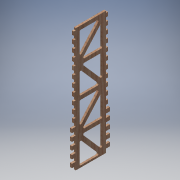
# Autodesk Inventor part: CrossBar4Alt
Saved by Autodesk Inventor 2019 (Build 230136000, 136)
## iProperties
Created: 2019-01-14
Part Number: CrossBar4Alt
Material: Wood (Birch)
Document SubType Name: Modeling
Designer: nxgam
Density: 0.55 g/cm^3
Appearance: Birch - Natural Polished
Author: nxgam
Autodesk Inventor part; units mm, degrees
ref_plane "YZ Plane" through (0, 0, 0) normal (1, 0, 0) x (0, 1, 0)
ref_plane "XZ Plane" through (0, 0, 0) normal (0, 1, 0) x (-1, 0, 0)
ref_plane "XY Plane" through (0, 0, 0) normal (0, 0, 1) x (1, 0, 0)
sketch "Sketch1" plane through (0, 0, 0) normal (1, 0, 0) x (0, 1, 0)
  line L0 (0, 0) -> (81.28, 0)
  line L1 (81.28, 0) -> (81.28, -91.44) construction
  line L2 (81.28, -91.44) -> (0, -91.44)
  line L3 (0, -91.44) -> (0, 0)
  line L4 (0, 0) -> (10.16, 0)
  line L5 (10.16, 0) -> (10.16, -5.08)
  line L6 (10.16, -5.08) -> (0, -5.08)
  line L7 (0, -5.08) -> (0, 0)
  line L8 (20.32, 0) -> (30.48, 0)
  line L9 (30.48, 0) -> (30.48, -5.08)
  line L10 (30.48, -5.08) -> (20.32, -5.08)
  line L11 (20.32, -5.08) -> (20.32, 0)
  line L12 (40.64, 0) -> (50.8, 0)
  line L13 (50.8, 0) -> (50.8, -5.08)
  line L14 (50.8, -5.08) -> (40.64, -5.08)
  line L15 (40.64, -5.08) -> (40.64, 0)
  line L16 (60.96, 0) -> (71.12, 0)
  line L17 (71.12, 0) -> (71.12, -5.08)
  line L18 (71.12, -5.08) -> (60.96, -5.08)
  line L19 (60.96, -5.08) -> (60.96, 0)
  line L20 (81.28, -45.72) -> (0, -45.72) construction
  line L21 (0, -91.44) -> (81.28, -91.44)
  line L22 (0, -91.44) -> (10.16, -91.44)
  line L23 (10.16, -91.44) -> (10.16, -86.36)
  line L24 (10.16, -86.36) -> (0, -86.36)
  line L25 (0, -86.36) -> (0, -91.44)
  line L26 (20.32, -91.44) -> (30.48, -91.44)
  line L27 (30.48, -91.44) -> (30.48, -86.36)
  line L28 (30.48, -86.36) -> (20.32, -86.36)
  line L29 (20.32, -86.36) -> (20.32, -91.44)
  line L30 (40.64, -91.44) -> (50.8, -91.44)
  line L31 (50.8, -91.44) -> (50.8, -86.36)
  line L32 (50.8, -86.36) -> (40.64, -86.36)
  line L33 (40.64, -86.36) -> (40.64, -91.44)
  line L34 (60.96, -91.44) -> (71.12, -91.44)
  line L35 (71.12, -91.44) -> (71.12, -86.36)
  line L36 (71.12, -86.36) -> (60.96, -86.36)
  line L37 (60.96, -86.36) -> (60.96, -91.44)
  line L38 (81.28, -86.36) -> (81.28, -91.44)
  line L39 (0, 0) -> (91.44, 0) construction
  line L40 (0, -91.44) -> (0, 0) construction
  line L41 (81.28, -10.16) -> (0, -10.16) construction
  line L42 (0, -10.16) -> (0, -81.28) construction
  line L43 (0, -81.28) -> (81.28, -81.28) construction
  line L44 (81.28, -81.28) -> (81.28, -10.16) construction
  line L45 (81.28, -10.16) -> (0, -81.28) construction
  line L46 (76.2, -28.3521) -> (76.2, -73.025)
  line L47 (73.025, -76.2) -> (21.9703, -76.2)
  line L48 (19.8795, -70.6356) -> (70.9342, -25.9627)
  arc A0 (76.2, -28.3521) -> (70.9342, -25.9627) centre (73.025, -28.3521) ccw
  arc A1 (73.025, -76.2) -> (76.2, -73.025) centre (73.025, -73.025) ccw
  arc A2 (19.8795, -70.6356) -> (21.9703, -76.2) centre (21.9703, -73.025) ccw
  line L49 (8.255, -15.24) -> (59.3097, -15.24)
  line L50 (61.4005, -20.8044) -> (10.3458, -65.4773)
  line L51 (5.08, -63.0879) -> (5.08, -18.415)
  arc A3 (61.4005, -20.8044) -> (59.3097, -15.24) centre (59.3097, -18.415) ccw
  arc A4 (5.08, -63.0879) -> (10.3458, -65.4773) centre (8.255, -63.0879) ccw
  arc A5 (8.255, -15.24) -> (5.08, -18.415) centre (8.255, -18.415) ccw
  line L52 (81.28, -45.72) -> (162.56, -45.72) construction
  line L53 (81.28, -10.16) -> (162.56, -10.16) construction
  line L54 (162.56, -81.28) -> (81.28, -81.28) construction
  line L55 (81.28, -10.16) -> (162.56, -81.28) construction
  line L56 (86.36, -28.3521) -> (86.36, -73.025)
  line L57 (89.535, -76.2) -> (140.5897, -76.2)
  line L58 (142.6805, -70.6356) -> (91.6258, -25.9627)
  arc A6 (91.6258, -25.9627) -> (86.36, -28.3521) centre (89.535, -28.3521) ccw
  arc A7 (86.36, -73.025) -> (89.535, -76.2) centre (89.535, -73.025) ccw
  arc A8 (140.5897, -76.2) -> (142.6805, -70.6356) centre (140.5897, -73.025) ccw
  line L59 (154.305, -15.24) -> (103.2503, -15.24)
  line L60 (101.1595, -20.8044) -> (152.2142, -65.4773)
  line L61 (157.48, -63.0879) -> (157.48, -18.415)
  arc A9 (103.2503, -15.24) -> (101.1595, -20.8044) centre (103.2503, -18.415) ccw
  arc A10 (152.2142, -65.4773) -> (157.48, -63.0879) centre (154.305, -63.0879) ccw
  arc A11 (157.48, -18.415) -> (154.305, -15.24) centre (154.305, -18.415) ccw
  line L62 (132.08, -86.36) -> (121.92, -86.36)
  line L63 (101.6, -86.36) -> (101.6, -91.44)
  line L64 (101.6, -91.44) -> (111.76, -91.44)
  line L65 (111.76, -91.44) -> (111.76, -86.36)
  line L66 (111.76, -86.36) -> (101.6, -86.36)
  line L67 (91.44, -86.36) -> (81.28, -86.36)
  line L68 (91.44, -91.44) -> (91.44, -86.36)
  line L69 (81.28, -91.44) -> (91.44, -91.44)
  line L70 (81.28, -91.44) -> (162.56, -91.44)
  line L71 (162.56, -91.44) -> (81.28, -91.44)
  line L72 (81.28, -81.28) -> (162.56, -81.28) construction
  line L73 (81.28, -10.16) -> (81.28, -81.28) construction
  line L74 (162.56, 0) -> (162.56, -91.44)
  line L75 (81.28, -91.44) -> (81.28, 0) construction
  line L76 (81.28, -91.44) -> (81.28, 0) construction
  line L77 (81.28, 0) -> (162.56, 0)
  line L78 (81.28, 0) -> (91.44, 0)
  line L79 (91.44, 0) -> (91.44, -5.08)
  line L80 (81.28, -5.08) -> (81.28, 0)
  line L81 (91.44, -5.08) -> (81.28, -5.08)
  line L82 (111.76, -5.08) -> (101.6, -5.08)
  line L83 (101.6, 0) -> (111.76, 0)
  line L84 (101.6, -5.08) -> (101.6, 0)
  line L85 (111.76, 0) -> (111.76, -5.08)
  line L86 (132.08, -5.08) -> (121.92, -5.08)
  line L87 (132.08, 0) -> (132.08, -5.08)
  line L88 (121.92, -5.08) -> (121.92, 0)
  line L89 (121.92, 0) -> (132.08, 0)
  line L90 (142.24, -5.08) -> (142.24, 0)
  line L91 (152.4, -5.08) -> (142.24, -5.08)
  line L92 (142.24, 0) -> (152.4, 0)
  line L93 (152.4, 0) -> (152.4, -5.08)
  line L94 (81.28, -86.36) -> (81.28, -91.44)
  line L95 (152.4, -86.36) -> (142.24, -86.36)
  line L96 (142.24, -91.44) -> (152.4, -91.44)
  line L97 (162.56, -86.36) -> (162.56, -91.44)
  line L98 (132.08, -91.44) -> (132.08, -86.36)
  line L99 (81.28, 0) -> (172.72, 0) construction
  line L100 (152.4, -91.44) -> (152.4, -86.36)
  line L101 (121.92, -86.36) -> (121.92, -91.44)
  line L102 (142.24, -86.36) -> (142.24, -91.44)
  line L103 (162.56, -81.28) -> (162.56, -10.16) construction
  line L104 (121.92, -91.44) -> (132.08, -91.44)
  line L105 (162.56, -10.16) -> (81.28, -10.16) construction
  line L106 (243.84, -81.28) -> (162.56, -81.28) construction
  line L107 (162.56, -45.72) -> (243.84, -45.72) construction
  line L108 (162.56, -10.16) -> (243.84, -81.28) construction
  line L109 (162.56, -10.16) -> (243.84, -10.16) construction
  line L110 (162.56, 0) -> (0, 0)
  line L111 (0, 0) -> (0, -91.44)
  line L112 (0, -91.44) -> (162.56, -91.44)
  line L113 (162.56, -91.44) -> (162.56, 0)
  line L114 (162.56, -91.44) -> (162.56, 0)
  line L115 (203.2, -86.36) -> (203.2, -91.44)
  line L116 (243.84, -45.72) -> (162.56, -45.72) construction
  line L117 (162.56, -81.28) -> (243.84, -81.28) construction
  line L118 (243.84, -10.16) -> (162.56, -81.28) construction
  line L119 (243.84, -10.16) -> (162.56, -10.16) construction
  line L120 (162.56, 0) -> (243.84, 0)
  line L121 (243.84, -91.44) -> (243.84, 0) construction
  line L122 (243.84, 0) -> (243.84, -91.44) construction
  line L123 (243.84, -91.44) -> (243.84, 0) construction
  line L124 (243.84, -91.44) -> (162.56, -91.44)
  line L125 (162.56, -91.44) -> (243.84, -91.44)
  line L126 (162.56, 0) -> (254, 0) construction
  line L127 (325.12, 0) -> (162.56, 0)
  line L128 (162.56, -91.44) -> (325.12, -91.44)
  line L129 (233.68, -91.44) -> (233.68, -86.36)
  line L130 (235.585, -76.2) -> (184.5303, -76.2)
  line L131 (223.52, -86.36) -> (223.52, -91.44)
  line L132 (243.84, -81.28) -> (243.84, -10.16) construction
  line L133 (193.04, 0) -> (193.04, -5.08)
  line L134 (193.04, -91.44) -> (193.04, -86.36)
  line L135 (193.04, -5.08) -> (182.88, -5.08)
  line L136 (193.04, -86.36) -> (182.88, -86.36)
  line L137 (182.88, -86.36) -> (182.88, -91.44)
  line L138 (172.72, 0) -> (172.72, -5.08)
  line L139 (162.56, -91.44) -> (162.56, 0) construction
  line L140 (162.56, 0) -> (172.72, 0)
  line L141 (162.56, -5.08) -> (162.56, 0)
  line L142 (162.56, -86.36) -> (162.56, -91.44)
  line L143 (172.72, -86.36) -> (162.56, -86.36)
  line L144 (172.72, -5.08) -> (162.56, -5.08)
  line L145 (162.56, -10.16) -> (162.56, -81.28) construction
  line L146 (223.52, -5.08) -> (223.52, 0)
  line L147 (233.68, -5.08) -> (223.52, -5.08)
  line L148 (223.52, 0) -> (233.68, 0)
  line L149 (233.68, 0) -> (233.68, -5.08)
  arc A12 (238.76, -28.3521) -> (233.4942, -25.9627) centre (235.585, -28.3521) ccw
  line L150 (182.88, -5.08) -> (182.88, 0)
  line L151 (254, -86.36) -> (243.84, -86.36)
  line L152 (264.16, -86.36) -> (264.16, -91.44)
  line L153 (264.16, -91.44) -> (274.32, -91.44)
  line L154 (294.64, -86.36) -> (284.48, -86.36)
  line L155 (316.865, -15.24) -> (265.8103, -15.24)
  line L156 (274.32, -86.36) -> (264.16, -86.36)
  line L157 (274.32, -91.44) -> (274.32, -86.36)
  line L158 (305.2405, -70.6356) -> (254.1858, -25.9627)
  arc A13 (248.92, -73.025) -> (252.095, -76.2) centre (252.095, -73.025) ccw
  line L159 (243.84, -10.16) -> (243.84, -81.28) construction
  arc A14 (265.8103, -15.24) -> (263.7195, -20.8044) centre (265.8103, -18.415) ccw
  line L160 (274.32, -5.08) -> (264.16, -5.08)
  line L161 (274.32, 0) -> (274.32, -5.08)
  line L162 (252.095, -76.2) -> (303.1497, -76.2)
  line L163 (263.7195, -20.8044) -> (314.7742, -65.4773)
  line L164 (325.12, -81.28) -> (243.84, -81.28) construction
  line L165 (243.84, -81.28) -> (325.12, -81.28) construction
  line L166 (243.84, -10.16) -> (325.12, -81.28) construction
  line L167 (243.84, -45.72) -> (325.12, -45.72) construction
  line L168 (243.84, -10.16) -> (325.12, -10.16) construction
  line L169 (325.12, -10.16) -> (243.84, -10.16) construction
  line L170 (243.84, 0) -> (325.12, 0)
  line L171 (243.84, 0) -> (335.28, 0) construction
  line L172 (320.04, -63.0879) -> (320.04, -18.415)
  line L173 (325.12, -91.44) -> (325.12, 0)
  line L174 (325.12, 0) -> (325.12, -91.44)
  arc A15 (314.7742, -65.4773) -> (320.04, -63.0879) centre (316.865, -63.0879) ccw
  line L175 (325.12, -91.44) -> (243.84, -91.44)
  line L176 (243.84, -91.44) -> (325.12, -91.44)
  line L177 (284.48, -86.36) -> (284.48, -91.44)
  line L178 (284.48, -91.44) -> (294.64, -91.44)
  line L179 (294.64, -91.44) -> (294.64, -86.36)
  line L180 (304.8, -86.36) -> (304.8, -91.44)
  line L181 (304.8, -91.44) -> (314.96, -91.44)
  line L182 (314.96, -91.44) -> (314.96, -86.36)
  arc A16 (303.1497, -76.2) -> (305.2405, -70.6356) centre (303.1497, -73.025) ccw
  line L183 (325.12, -86.36) -> (325.12, -91.44)
  line L184 (314.96, -86.36) -> (304.8, -86.36)
  line L185 (243.84, -86.36) -> (243.84, -91.44)
  arc A17 (235.585, -76.2) -> (238.76, -73.025) centre (235.585, -73.025) ccw
  line L186 (238.76, -28.3521) -> (238.76, -73.025)
  line L187 (223.52, -91.44) -> (233.68, -91.44)
  line L188 (203.2, -91.44) -> (213.36, -91.44)
  line L189 (213.36, -86.36) -> (203.2, -86.36)
  line L190 (172.72, -91.44) -> (172.72, -86.36)
  line L191 (248.92, -28.3521) -> (248.92, -73.025)
  line L192 (233.68, -86.36) -> (223.52, -86.36)
  line L193 (243.84, -86.36) -> (243.84, -91.44)
  line L194 (243.84, -91.44) -> (254, -91.44)
  line L195 (213.36, -91.44) -> (213.36, -86.36)
  line L196 (254, -91.44) -> (254, -86.36)
  line L197 (162.56, -91.44) -> (172.72, -91.44)
  line L198 (182.88, -91.44) -> (193.04, -91.44)
  line L199 (213.36, 0) -> (213.36, -5.08)
  line L200 (213.36, -5.08) -> (203.2, -5.08)
  line L201 (203.2, 0) -> (213.36, 0)
  line L202 (182.88, 0) -> (193.04, 0)
  line L203 (203.2, -5.08) -> (203.2, 0)
  line L204 (254, -5.08) -> (243.84, -5.08)
  line L205 (243.84, -5.08) -> (243.84, 0)
  line L206 (243.84, 0) -> (254, 0)
  line L207 (182.4395, -70.6356) -> (233.4942, -25.9627)
  arc A18 (254.1858, -25.9627) -> (248.92, -28.3521) centre (252.095, -28.3521) ccw
  line L208 (254, 0) -> (254, -5.08)
  line L209 (264.16, 0) -> (274.32, 0)
  line L210 (264.16, -5.08) -> (264.16, 0)
  line L211 (294.64, 0) -> (294.64, -5.08)
  line L212 (304.8, -5.08) -> (304.8, 0)
  line L213 (162.56, 0) -> (162.56, -91.44)
  arc A19 (223.9605, -20.8044) -> (221.8697, -15.24) centre (221.8697, -18.415) ccw
  arc A20 (182.4395, -70.6356) -> (184.5303, -76.2) centre (184.5303, -73.025) ccw
  line L214 (223.9605, -20.8044) -> (172.9058, -65.4773)
  line L215 (167.64, -63.0879) -> (167.64, -18.415)
  line L216 (170.815, -15.24) -> (221.8697, -15.24)
  arc A21 (170.815, -15.24) -> (167.64, -18.415) centre (170.815, -18.415) ccw
  arc A22 (167.64, -63.0879) -> (172.9058, -65.4773) centre (170.815, -63.0879) ccw
  line L217 (406.4, -81.28) -> (325.12, -81.28) construction
  line L218 (325.12, -45.72) -> (406.4, -45.72) construction
  line L219 (325.12, -10.16) -> (406.4, -81.28) construction
  line L220 (325.12, -10.16) -> (406.4, -10.16) construction
  line L221 (325.12, -81.28) -> (325.12, -10.16) construction
  arc A23 (320.04, -18.415) -> (316.865, -15.24) centre (316.865, -18.415) ccw
  line L222 (294.64, -5.08) -> (284.48, -5.08)
  line L223 (284.48, -5.08) -> (284.48, 0)
  line L224 (314.96, 0) -> (314.96, -5.08)
  line L225 (314.96, -5.08) -> (304.8, -5.08)
  line L226 (304.8, 0) -> (314.96, 0)
  line L227 (284.48, 0) -> (294.64, 0)
  point P0 (40.64, -45.72)
  point P1 (121.92, -45.72)
  point P2 (81.28, -45.72)
  point P3 (203.2, -45.72)
  point P4 (203.2, -45.72)
  point P5 (284.48, -45.72)
  point P6 (365.76, -45.72)
  dimension "d0" = 81.28
  dimension "d1" = 91.44
  dimension "d2" = 10.16
  dimension "d3" = 5.08
  dimension "d6" = 20.32
  dimension "d12" = 5.08
  dimension "d13" = 0
  dimension "d14" = 3.175
  dimension "d15" = 3.175
  dimension "d16" = 10.16
  dimension "d17" = 10.16
  dimension "d18" = 5.08
  dimension "d20" = 10.16
  dimension "d21" = 5.08
  dimension "d26" = 81.28
  dimension "d38" = 162.56
  constraints: 456 end point, 48 point on circle, 38 symmetric about line, 24 centre point, 12 tangent, 10 parallel, 8 horizontal, 5 midpoint, 5 perpendicular, 4 equal radius, 2 coincident, 2 collinear, 2 point on line, 393 other
  measures "d0" distance of L1.end L2.end
  measures "d1" distance of L0.end L1.end
  measures "d2" distance of L5.end L6.end
  measures "d3" distance of L4.end L5.end
  measures "d6" distance of L0.start L8.start
  measures "d12" distance between parallel lines of L28 L43
  measures "d13" distance between parallel lines of L44 L1
  measures "d14" radius of A0
  measures "d15" radius of A3
  measures "d16" distance between parallel lines of L50 L48
  measures "d17" distance between parallel lines of L28 L47
  measures "d18" distance between parallel lines of L3 L51
  measures "d20" distance between parallel lines of L14 L49
  measures "d21" distance between parallel lines of L1 L46
  measures "d26" distance of L32.start L62.start
  measures "d38" distance of L2.end L114.start
extrude "Extrusion2" add sketch "Sketch1" along normal blind 5.08 contours L0 L11 L10 L9 L15 L14 L13 L19 L18 L17 L80 L81 L79 L77 L84 L82 L85 L88 L86 L87 L90 L91 L93 L74 L70 L100 L95 L102 L98 L62 L101 L65 L66 L63 L68 L67 L38 L2 L35 L36 L37 L31 L32 L33 L27 L28 L29 L23 L24 L3 L6 L5
extrude "Extrusion3" add sketch "Sketch1" along normal blind 5.08 contours L144 L138 L120 L150 L135 L133 L203 L200 L199 L146 L147 L149 L205 L204 L208 L127 L210 L160 L161 L223 L222 L211 L212 L225 L224 L173 L128 L182 L184 L180 L179 L154 L177 L157 L156 L152 L196 L151 L185 L124 L129 L192 L131 L195 L189 L115 L134 L136 L137 L190 L143 L74
thicken "Thicken1" [suppressed]
sketch "Sketch2" plane through (0, 325.12, 0) normal (0, 1, 0) x (1, 0, 0)
  line L0 (0, 91.44) -> (0, 0) projected
  line L1 (0, 0) -> (5.08, 0) projected
  line L2 (5.08, 91.44) -> (5.08, 0) projected
  line L3 (0, 91.44) -> (5.08, 91.44) projected
  line L4 (5.08, 5.08) -> (0, 5.08) projected
  line L5 (5.08, 91.44) -> (5.08, 86.36) projected
  line L6 (0, 5.08) -> (5.08, 5.08)
  line L7 (5.08, 5.08) -> (5.08, 86.36)
  line L8 (5.08, 86.36) -> (0, 86.36)
  line L9 (0, 86.36) -> (0, 5.08)
  constraints: 8 end point, 2 parallel, 1 horizontal, 1 perpendicular
extrude "Extrusion4" add sketch "Sketch2" along normal blind 5.08 contours L8 L2 L4 L0
sketch "Sketch3" plane through (5.08, 0, 0) normal (1, 0, 0) x (0, 0, -1)
  arc A0 (63.0879, 167.64) -> (65.4773, 172.9058) centre (63.0879, 170.815) ccw projected
  line L0 (63.0879, 167.64) -> (18.415, 167.64) projected
  arc A1 (15.24, 170.815) -> (18.415, 167.64) centre (18.415, 170.815) ccw projected
  line L1 (15.24, 170.815) -> (15.24, 221.8697) projected
  arc A2 (20.8044, 223.9605) -> (15.24, 221.8697) centre (18.415, 221.8697) ccw projected
  line L2 (20.8044, 223.9605) -> (65.4773, 172.9058) projected
  arc A3 (70.6356, 182.4395) -> (76.2, 184.5303) centre (73.025, 184.5303) ccw projected
  line L3 (70.6356, 182.4395) -> (25.9627, 233.4942) projected
  arc A4 (28.3521, 238.76) -> (25.9627, 233.4942) centre (28.3521, 235.585) ccw projected
  line L4 (28.3521, 238.76) -> (73.025, 238.76) projected
  arc A5 (76.2, 235.585) -> (73.025, 238.76) centre (73.025, 235.585) ccw projected
  line L5 (76.2, 235.585) -> (76.2, 184.5303) projected
  arc A6 (76.2, 303.1497) -> (70.6356, 305.2405) centre (73.025, 303.1497) ccw projected
  line L6 (76.2, 303.1497) -> (76.2, 252.095) projected
  arc A7 (73.025, 248.92) -> (76.2, 252.095) centre (73.025, 252.095) ccw projected
  line L7 (73.025, 248.92) -> (28.3521, 248.92) projected
  arc A8 (25.9627, 254.1858) -> (28.3521, 248.92) centre (28.3521, 252.095) ccw projected
  line L8 (25.9627, 254.1858) -> (70.6356, 305.2405) projected
  arc A9 (18.415, 320.04) -> (15.24, 316.865) centre (18.415, 316.865) ccw projected
  line L9 (18.415, 320.04) -> (63.0879, 320.04) projected
  arc A10 (65.4773, 314.7742) -> (63.0879, 320.04) centre (63.0879, 316.865) ccw projected
  line L10 (65.4773, 314.7742) -> (20.8044, 263.7195) projected
  arc A11 (15.24, 265.8103) -> (20.8044, 263.7195) centre (18.415, 265.8103) ccw projected
  line L11 (15.24, 265.8103) -> (15.24, 316.865) projected
  arc A12 (73.025, 86.36) -> (76.2, 89.535) centre (73.025, 89.535) ccw projected
  line L12 (73.025, 86.36) -> (28.3521, 86.36) projected
  arc A13 (25.9627, 91.6258) -> (28.3521, 86.36) centre (28.3521, 89.535) ccw projected
  line L13 (25.9627, 91.6258) -> (70.6356, 142.6805) projected
  arc A14 (76.2, 140.5897) -> (70.6356, 142.6805) centre (73.025, 140.5897) ccw projected
  line L14 (76.2, 140.5897) -> (76.2, 89.535) projected
  arc A15 (15.24, 103.2503) -> (20.8044, 101.1595) centre (18.415, 103.2503) ccw projected
  line L15 (15.24, 103.2503) -> (15.24, 154.305) projected
  arc A16 (18.415, 157.48) -> (15.24, 154.305) centre (18.415, 154.305) ccw projected
  line L16 (18.415, 157.48) -> (63.0879, 157.48) projected
  arc A17 (65.4773, 152.2142) -> (63.0879, 157.48) centre (63.0879, 154.305) ccw projected
  line L17 (65.4773, 152.2142) -> (20.8044, 101.1595) projected
  arc A18 (28.3521, 76.2) -> (25.9627, 70.9342) centre (28.3521, 73.025) ccw projected
  line L18 (28.3521, 76.2) -> (73.025, 76.2) projected
  arc A19 (76.2, 73.025) -> (73.025, 76.2) centre (73.025, 73.025) ccw projected
  line L19 (76.2, 73.025) -> (76.2, 21.9703) projected
  arc A20 (70.6356, 19.8795) -> (76.2, 21.9703) centre (73.025, 21.9703) ccw projected
  line L20 (70.6356, 19.8795) -> (25.9627, 70.9342) projected
  arc A21 (20.8044, 61.4005) -> (15.24, 59.3097) centre (18.415, 59.3097) ccw projected
  line L21 (20.8044, 61.4005) -> (65.4773, 10.3458) projected
  arc A22 (63.0879, 5.08) -> (65.4773, 10.3458) centre (63.0879, 8.255) ccw projected
  line L22 (63.0879, 5.08) -> (18.415, 5.08) projected
  arc A23 (15.24, 8.255) -> (18.415, 5.08) centre (18.415, 8.255) ccw projected
  line L23 (15.24, 8.255) -> (15.24, 59.3097) projected
  line L24 (91.44, 142.24) -> (86.36, 142.24) projected
  line L25 (86.36, 142.24) -> (86.36, 152.4) projected
  line L26 (86.36, 152.4) -> (91.44, 152.4) projected
  line L27 (91.44, 152.4) -> (91.44, 162.56) projected
  line L28 (91.44, 162.56) -> (86.36, 162.56) projected
  line L29 (86.36, 162.56) -> (86.36, 172.72) projected
  line L30 (86.36, 172.72) -> (91.44, 172.72) projected
  line L31 (91.44, 172.72) -> (91.44, 182.88) projected
  line L32 (91.44, 182.88) -> (86.36, 182.88) projected
  line L33 (86.36, 182.88) -> (86.36, 193.04) projected
  line L34 (86.36, 193.04) -> (91.44, 193.04) projected
  line L35 (91.44, 193.04) -> (91.44, 203.2) projected
  line L36 (91.44, 203.2) -> (86.36, 203.2) projected
  line L37 (86.36, 203.2) -> (86.36, 213.36) projected
  line L38 (86.36, 213.36) -> (91.44, 213.36) projected
  line L39 (91.44, 213.36) -> (91.44, 223.52) projected
  line L40 (91.44, 223.52) -> (86.36, 223.52) projected
  line L41 (86.36, 223.52) -> (86.36, 233.68) projected
  line L42 (86.36, 233.68) -> (91.44, 233.68) projected
  line L43 (91.44, 233.68) -> (91.44, 243.84) projected
  line L44 (91.44, 243.84) -> (86.36, 243.84) projected
  line L45 (86.36, 243.84) -> (86.36, 254) projected
  line L46 (86.36, 254) -> (91.44, 254) projected
  line L47 (91.44, 254) -> (91.44, 264.16) projected
  line L48 (91.44, 264.16) -> (86.36, 264.16) projected
  line L49 (86.36, 264.16) -> (86.36, 274.32) projected
  line L50 (86.36, 274.32) -> (91.44, 274.32) projected
  line L51 (91.44, 274.32) -> (91.44, 284.48) projected
  line L52 (91.44, 284.48) -> (86.36, 284.48) projected
  line L53 (86.36, 284.48) -> (86.36, 294.64) projected
  line L54 (86.36, 294.64) -> (91.44, 294.64) projected
  line L55 (91.44, 294.64) -> (91.44, 304.8) projected
  line L56 (91.44, 304.8) -> (86.36, 304.8) projected
  line L57 (86.36, 304.8) -> (86.36, 314.96) projected
  line L58 (86.36, 314.96) -> (91.44, 314.96) projected
  line L59 (91.44, 314.96) -> (91.44, 325.12) projected
  line L60 (91.44, 325.12) -> (86.36, 325.12) projected
  line L61 (86.36, 325.12) -> (86.36, 330.2) projected
  line L62 (5.08, 330.2) -> (86.36, 330.2) projected
  line L63 (5.08, 325.12) -> (5.08, 330.2) projected
  line L64 (5.08, 325.12) -> (0, 325.12) projected
  line L65 (0, 325.12) -> (0, 314.96) projected
  line L66 (0, 314.96) -> (5.08, 314.96) projected
  line L67 (5.08, 314.96) -> (5.08, 304.8) projected
  line L68 (5.08, 304.8) -> (0, 304.8) projected
  line L69 (0, 304.8) -> (0, 294.64) projected
  line L70 (0, 294.64) -> (5.08, 294.64) projected
  line L71 (5.08, 294.64) -> (5.08, 284.48) projected
  line L72 (5.08, 284.48) -> (0, 284.48) projected
  line L73 (0, 284.48) -> (0, 274.32) projected
  line L74 (0, 274.32) -> (5.08, 274.32) projected
  line L75 (5.08, 274.32) -> (5.08, 264.16) projected
  line L76 (5.08, 264.16) -> (0, 264.16) projected
  line L77 (0, 264.16) -> (0, 254) projected
  line L78 (0, 254) -> (5.08, 254) projected
  line L79 (5.08, 254) -> (5.08, 243.84) projected
  line L80 (5.08, 243.84) -> (0, 243.84) projected
  line L81 (0, 243.84) -> (0, 233.68) projected
  line L82 (0, 233.68) -> (5.08, 233.68) projected
  line L83 (5.08, 233.68) -> (5.08, 223.52) projected
  line L84 (5.08, 223.52) -> (0, 223.52) projected
  line L85 (0, 223.52) -> (0, 213.36) projected
  line L86 (0, 213.36) -> (5.08, 213.36) projected
  line L87 (5.08, 213.36) -> (5.08, 203.2) projected
  line L88 (5.08, 203.2) -> (0, 203.2) projected
  line L89 (0, 203.2) -> (0, 193.04) projected
  line L90 (0, 193.04) -> (5.08, 193.04) projected
  line L91 (5.08, 193.04) -> (5.08, 182.88) projected
  line L92 (5.08, 182.88) -> (0, 182.88) projected
  line L93 (0, 182.88) -> (0, 172.72) projected
  line L94 (0, 172.72) -> (5.08, 172.72) projected
  line L95 (5.08, 172.72) -> (5.08, 162.56) projected
  line L96 (5.08, 162.56) -> (0, 162.56) projected
  line L97 (0, 162.56) -> (0, 152.4) projected
  line L98 (0, 152.4) -> (5.08, 152.4) projected
  line L99 (5.08, 152.4) -> (5.08, 142.24) projected
  line L100 (5.08, 142.24) -> (0, 142.24) projected
  line L101 (0, 142.24) -> (0, 132.08) projected
  line L102 (0, 132.08) -> (5.08, 132.08) projected
  line L103 (5.08, 132.08) -> (5.08, 121.92) projected
  line L104 (5.08, 121.92) -> (0, 121.92) projected
  line L105 (0, 121.92) -> (0, 111.76) projected
  line L106 (0, 111.76) -> (5.08, 111.76) projected
  line L107 (5.08, 111.76) -> (5.08, 101.6) projected
  line L108 (5.08, 101.6) -> (0, 101.6) projected
  line L109 (0, 101.6) -> (0, 91.44) projected
  line L110 (0, 91.44) -> (5.08, 91.44) projected
  line L111 (5.08, 91.44) -> (5.08, 81.28) projected
  line L112 (5.08, 81.28) -> (0, 81.28) projected
  line L113 (0, 81.28) -> (0, 71.12) projected
  line L114 (0, 71.12) -> (5.08, 71.12) projected
  line L115 (5.08, 71.12) -> (5.08, 60.96) projected
  line L116 (5.08, 60.96) -> (0, 60.96) projected
  line L117 (0, 60.96) -> (0, 50.8) projected
  line L118 (0, 50.8) -> (5.08, 50.8) projected
  line L119 (5.08, 50.8) -> (5.08, 40.64) projected
  line L120 (5.08, 40.64) -> (0, 40.64) projected
  line L121 (0, 40.64) -> (0, 30.48) projected
  line L122 (0, 30.48) -> (5.08, 30.48) projected
  line L123 (5.08, 30.48) -> (5.08, 20.32) projected
  line L124 (5.08, 20.32) -> (0, 20.32) projected
  line L125 (0, 20.32) -> (0, 10.16) projected
  line L126 (0, 10.16) -> (5.08, 10.16) projected
  line L127 (5.08, 10.16) -> (5.08, 0) projected
  line L128 (5.08, 0) -> (86.36, 0) projected
  line L129 (86.36, 0) -> (86.36, 10.16) projected
  line L130 (86.36, 10.16) -> (91.44, 10.16) projected
  line L131 (91.44, 10.16) -> (91.44, 20.32) projected
  line L132 (91.44, 20.32) -> (86.36, 20.32) projected
  line L133 (86.36, 20.32) -> (86.36, 30.48) projected
  line L134 (86.36, 30.48) -> (91.44, 30.48) projected
  line L135 (91.44, 30.48) -> (91.44, 40.64) projected
  line L136 (91.44, 40.64) -> (86.36, 40.64) projected
  line L137 (86.36, 40.64) -> (86.36, 50.8) projected
  line L138 (86.36, 50.8) -> (91.44, 50.8) projected
  line L139 (91.44, 50.8) -> (91.44, 60.96) projected
  line L140 (91.44, 60.96) -> (86.36, 60.96) projected
  line L141 (86.36, 60.96) -> (86.36, 71.12) projected
  line L142 (86.36, 71.12) -> (91.44, 71.12) projected
  line L143 (91.44, 71.12) -> (91.44, 81.28) projected
  line L144 (91.44, 81.28) -> (86.36, 81.28) projected
  line L145 (86.36, 81.28) -> (86.36, 91.44) projected
  line L146 (86.36, 91.44) -> (91.44, 91.44) projected
  line L147 (91.44, 91.44) -> (91.44, 101.6) projected
  line L148 (91.44, 101.6) -> (86.36, 101.6) projected
  line L149 (86.36, 101.6) -> (86.36, 111.76) projected
  line L150 (86.36, 111.76) -> (91.44, 111.76) projected
  line L151 (91.44, 111.76) -> (91.44, 121.92) projected
  line L152 (91.44, 121.92) -> (86.36, 121.92) projected
  line L153 (86.36, 121.92) -> (86.36, 132.08) projected
  line L154 (86.36, 132.08) -> (91.44, 132.08) projected
  line L155 (91.44, 132.08) -> (91.44, 142.24) projected
  line L156 (0, 10.16) -> (-5.08, 10.16)
  line L157 (-5.08, 10.16) -> (-5.08, 20.32)
  line L158 (-5.08, 20.32) -> (0, 20.32)
  line L159 (0, 20.32) -> (0, 10.16)
  line L160 (91.44, 10.16) -> (96.52, 10.16)
  line L161 (96.52, 10.16) -> (96.52, 20.32)
  line L162 (96.52, 20.32) -> (91.44, 20.32)
  line L163 (91.44, 20.32) -> (91.44, 10.16)
  line L164 (5.08, 20.32) -> (0, 20.32) projected
  line L165 (91.44, 40.64) -> (91.44, 30.48)
  line L166 (91.44, 30.48) -> (96.52, 30.48)
  line L167 (96.52, 30.48) -> (96.52, 40.64)
  line L168 (96.52, 40.64) -> (91.44, 40.64)
  line L169 (-5.08, 40.64) -> (0, 40.64)
  line L170 (0, 30.48) -> (-5.08, 30.48)
  line L171 (-5.08, 30.48) -> (-5.08, 40.64)
  line L172 (0, 40.64) -> (0, 30.48)
  line L173 (91.44, 60.96) -> (91.44, 50.8)
  line L174 (91.44, 50.8) -> (96.52, 50.8)
  line L175 (96.52, 50.8) -> (96.52, 60.96)
  line L176 (96.52, 60.96) -> (91.44, 60.96)
  line L177 (-5.08, 60.96) -> (0, 60.96)
  line L178 (0, 50.8) -> (-5.08, 50.8)
  line L179 (-5.08, 50.8) -> (-5.08, 60.96)
  line L180 (0, 60.96) -> (0, 50.8)
  line L181 (91.44, 81.28) -> (91.44, 71.12)
  line L182 (91.44, 71.12) -> (96.52, 71.12)
  line L183 (96.52, 71.12) -> (96.52, 81.28)
  line L184 (96.52, 81.28) -> (91.44, 81.28)
  line L185 (-5.08, 81.28) -> (0, 81.28)
  line L186 (0, 71.12) -> (-5.08, 71.12)
  line L187 (-5.08, 71.12) -> (-5.08, 81.28)
  line L188 (0, 81.28) -> (0, 71.12)
  line L189 (91.44, 101.6) -> (91.44, 91.44)
  line L190 (91.44, 91.44) -> (96.52, 91.44)
  line L191 (96.52, 91.44) -> (96.52, 101.6)
  line L192 (96.52, 101.6) -> (91.44, 101.6)
  line L193 (-5.08, 101.6) -> (0, 101.6)
  line L194 (0, 91.44) -> (-5.08, 91.44)
  line L195 (-5.08, 91.44) -> (-5.08, 101.6)
  line L196 (0, 101.6) -> (0, 91.44)
  point P0 (0, 0)
  point P1 (0, 40.64)
  point P2 (0, 60.96)
  point P3 (0, 81.28)
  point P4 (0, 101.6)
  dimension "d46" = 5.08
  dimension "d47" = 5.08
  dimension "d50" = 20.32
  constraints: 80 end point, 5 point on line, 4 parallel, 2 horizontal, 2 perpendicular, 1 collinear, 1 vertical, 72 other
  measures "d46" distance of L161.end L162.end
  measures "d47" distance of L125.end L156.end
  measures "d50" distance of L130.end L165.end
extrude "Extrusion5" add sketch "Sketch3" against normal blind 5.08 contours L192 L191 L190 L147 | L184 L183 L182 L143 | L176 L175 L174 L139 | L168 L167 L166 L135 | L162 L161 L160 L131 | L156 L157 L158 L125 | L170 L171 L169 L121 | L178 L179 L177 L117 | L186 L187 L185 L113 | L194 L195 L193 L109
equation "\"d16\" = d17"
equation "\"d18\" = d21"
equation "\"d20\" = d17"
equation "\"d26\" = d0"
equation "\"d38\" = 2 * d0"
equation "\"d47\" = d46"
body "Solid2"
